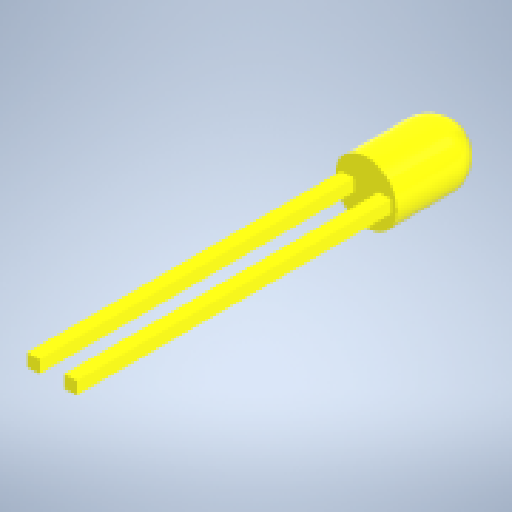
# Autodesk Inventor part: LED
Saved by Autodesk Inventor 2023.1 (Build 271208000, 208)
## iProperties
Created: 2022-07-14
Part Number: LED
Material: PC/ABS Plastic
Document SubType Name: Modeling
Designer: Eli
Density: 0.357273 g/cm^3
Appearance: Smooth - Yellow
Author: Eli
Autodesk Inventor part; units mm, degrees
ref_plane "YZ Plane" through (0, 0, 0) normal (1, 0, 0) x (0, 1, 0)
ref_plane "XZ Plane" through (0, 0, 0) normal (0, 1, 0) x (-1, 0, 0)
ref_plane "XY Plane" through (0, 0, 0) normal (0, 0, 1) x (1, 0, 0)
sketch "Sketch1" plane through (0, 0, 0) normal (1, 0, 0) x (0, 1, 0)
  line L0 (2.5, 0) -> (-2.5, 0)
  line L1 (-2.5, 0) -> (-2.5, -5.1)
  line L2 (-2.5, -5.1) -> (2.5, -5.1)
  line L3 (2.5, -5.1) -> (2.5, 0)
  circle A0 centre (0, -5.1) radius 2.5
  line L4 (0, 0) -> (0, -7.6)
  dimension "d0" = 5
  dimension "d1" = 5.1
  constraints: 10 end point, 3 perpendicular, 2 coincident, 2 midpoint, 2 point on circle, 1 centre point, 1 horizontal, 1 vertical
  measures "d0" distance of L0.start L0.end
  measures "d1" distance of L2.end L0.start
revolve "Revolution1" add sketch "Sketch1" angle 360 about axis through (0, 0, 0) along (0, 0, -1) picked at (1.6458, -5.2854) picked at (1.6458, -4.9146) contours L3 A0 L4 L0 | A0 L4 L2 | L2 L4 A0
sketch "Sketch2" plane through (0, 0, 0) normal (0, 0, 1) x (1, 0, 0)
  line L0 (-1, -0.5) -> (-2, -0.5)
  line L1 (-2, -0.5) -> (-2, 0.5)
  line L2 (-2, 0.5) -> (-1, 0.5)
  line L3 (-1, 0.5) -> (-1, -0.5)
  line L4 (2, -0.5) -> (1, -0.5)
  line L5 (1, -0.5) -> (1, 0.5)
  line L6 (1, 0.5) -> (2, 0.5)
  line L7 (2, 0.5) -> (2, -0.5)
  point P0 (0, 0)
  point P1 (1, 0)
  dimension "d3" = 1
  dimension "d4" = 1
  dimension "d5" = 1
  dimension "d6" = 2
  dimension "d7" = 1
  constraints: 16 end point, 4 parallel, 2 horizontal, 2 perpendicular, 2 point on line, 1 horizontal alignment, 1 midpoint
  measures "d3" distance of L1.end L2.end
  measures "d4" distance of L2.end L0.start
  measures "d5" distance of L5.end L6.end
  measures "d6" distance of L2.end L5.end
  measures "d7" horizontal distance of point (0, 0) L0.start
extrude "Extrusion1" add sketch "Sketch2" along normal blind 25.4
body "Solid1"
